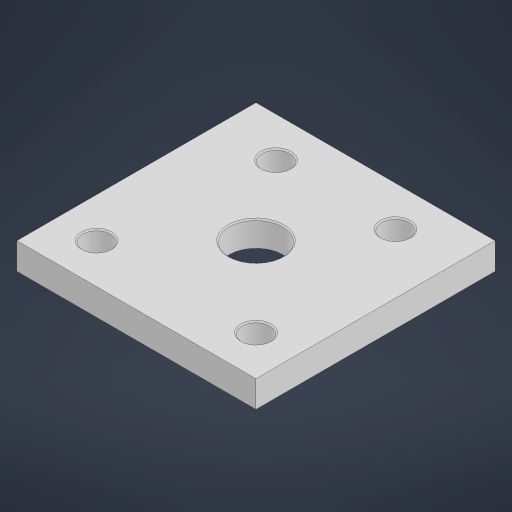
# Autodesk Inventor part: AP1-002
Saved by Autodesk Inventor 2024.3 (Build 283343000, 343)
## iProperties
Created: 2024-05-02
Part Number: AP1-002
Material: Generic
Document SubType Name: Modeling
Designer: fablabadmin
Density: 1 g/cm^3
Appearance: Default
Description: Plate top
Author: fablabadmin
Autodesk Inventor part; units mm, degrees
ref_plane "YZ Plane" through (0, 0, 0) normal (1, 0, 0) x (0, 1, 0)
ref_plane "XZ Plane" through (0, 0, 0) normal (0, 1, 0) x (-1, 0, 0)
ref_plane "XY Plane" through (0, 0, 0) normal (0, 0, 1) x (1, 0, 0)
sketch "Sketch1" plane through (0, 0, 0) normal (0, 1, 0) x (-1, 0, 0)
  line L0 (-45, 45) -> (45, 45)
  line L1 (45, 45) -> (45, -45)
  line L2 (45, -45) -> (-45, -45)
  line L3 (-45, -45) -> (-45, 45)
  line L4 (-45, 45) -> (45, -45) construction
  line L5 (45, 45) -> (-45, -45) construction
  line L6 (-30, 30) -> (30, 30) construction
  line L7 (30, 30) -> (30, -30) construction
  line L8 (30, -30) -> (-30, -30) construction
  line L9 (-30, -30) -> (-30, 30) construction
  line L10 (-30, 30) -> (30, -30) construction
  line L11 (30, 30) -> (-30, -30) construction
  line L12 (-22.5, 30) -> (22.5, 30) construction
  line L13 (22.5, 30) -> (22.5, -30) construction
  line L14 (22.5, -30) -> (-22.5, -30) construction
  line L15 (-22.5, -30) -> (-22.5, 30) construction
  line L16 (-22.5, 30) -> (22.5, -30) construction
  line L17 (22.5, 30) -> (-22.5, -30) construction
  circle A0 centre (0, 0) radius 10
  dimension "d0" = 90
  dimension "d1" = 60
  dimension "d2" = 45
  dimension "d3" = 20
  constraints: 36 end point, 6 midpoint, 6 parallel, 5 coincident, 5 perpendicular, 3 horizontal, 1 centre point, 1 point on line
  measures "d0" distance of L1.end L2.end
  measures "d1" distance of L7.end L8.end
  measures "d2" distance between parallel lines of L15 L13
  measures "d3" diameter of A0
extrude "Extrusion1" add sketch "Sketch1" against normal blind 10
hole "Hole1" at (-22.5, 0, -30) at (22.5, 0, -30) at (-30, 0, 30) at (30, 0, 30) direction (0, -1, 0) diameter 10.5 end through all
chamfer "Chamfer1" distance 0.5 angle 45 10 edges at (-22.5, 0, -35.25) (22.5, -10, -35.25) (22.5, 0, -35.25) (30, 0, 24.75) (30, -10, 24.75) (-30, 0, 24.75) (-30, -10, 24.75) (-22.5, -10, -35.25) (10, 0, 0) (10, -10, 0)
body "Solid1"
